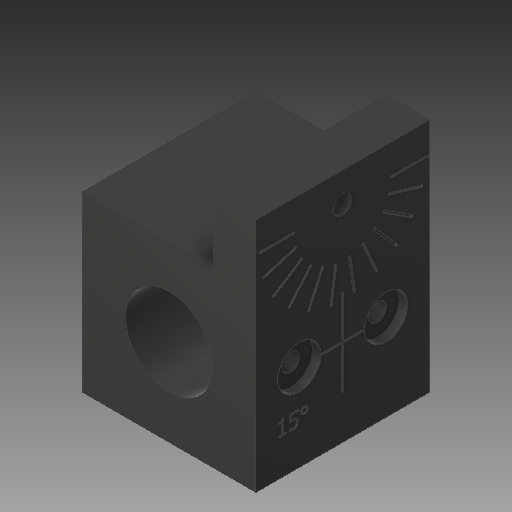
# Autodesk Inventor part: cam_holder_end_part
Saved by Autodesk Inventor 2019 (Build 230136000, 136)
## iProperties
Created: 2024-08-06
Part Number: cam_holder_end_part
Material: Acetalharz, Schwarz
Document SubType Name: Modeling
Designer: nic
Density: 1.425 g/cm^3
Appearance: Glatt - Schwarz
Author: nic
Autodesk Inventor part; units mm, degrees
ref_plane "YZ Plane" through (0, 0, 0) normal (1, 0, 0) x (0, 1, 0)
ref_plane "XY Plane" through (0, 0, 0) normal (0, 0, 1) x (1, 0, 0)
sketch "Skizze1" plane through (0, 0, 0) normal (0, 0, 1) x (1, 0, 0)
  circle A0 centre (0, 0) radius 10.05
  circle A1 centre (0, 0) radius 20
  line L0 (20, 0) -> (10.05, 0)
  line L1 (10.05, 0) -> (10.05, 35)
  line L2 (10.05, 35) -> (20, 35)
  line L3 (20, 35) -> (20, 0)
  dimension "d1" = 40
  dimension "d0" = 20.1
  dimension "d2" = 35
  constraints: 8 end point, 2 coincident, 2 parallel, 1 centre point, 1 horizontal, 1 horizontal alignment, 1 perpendicular, 2 other
  measures "d0" diameter of A0
  measures "d2" distance of L0.end L1.end
extrude "Extrusion1" add sketch "Skizze1" along normal blind 40
sketch "Skizze3" plane through (10.05, 17.2915, 0) normal (-1, 0, 0) x (0, 0, 1)
  line L0 (0, 0) -> (40, 0) construction
  line L1 (40, 17.7085) -> (40, 0) construction
  line L2 (0, 17.7085) -> (40, 17.7085) construction
  line L3 (0, 0) -> (0, 17.7085) construction
  line L4 (0, 17.7085) -> (40, 17.7085) projected
  line L5 (20, 17.7085) -> (20, 7.753)
  line L6 (40, 17.7085) -> (40, 0) projected
  line L7 (40, 10.1178) -> (0, 10.1178)
  point P0 (0, -17.2915)
  point P1 (20, 10.1178)
  constraints: 4 end point, 2 midpoint, 2 point on line, 1 perpendicular, 1 vertical
hole "Bohrung1" at (10.05, 27.4094, 20) direction (1, 0, 0) diameter 4.2 depth 20 tip angle 118 counterbore diameter 8 counterbore depth 3 clearance for "Zylinderschraube mit Schlitz DIN 84" size "M4" standard "DIN"
ref_plane "Arbeitsebene1" through (0, -20, 0) normal (0, 1, 0) x (-1, 0, 0)
sketch "Skizze6" plane through (10.05, 17.2915, 0) normal (-1, 0, 0) x (0, 0, 1)
  circle A0 centre (20, 10.1178) radius 2.1 projected
  circle A1 centre (20, 10.1178) radius 4
  circle A2 centre (20, 10.1178) radius 2.05
  point P0 (0, -17.2915)
  dimension "d37" = 4.1
  constraints: 2 centre point, 2 coincident
  measures "d37" diameter of A2
extrude "Extrusion4" add sketch "Skizze6" against normal up to surface (3 mm away) contours A1
sketch "Skizze15" plane through (0, 0, 0) normal (0, 0, -1) x (-1, 0, 0)
  circle A0 centre (0, 0) radius 10.1
  dimension "d75" = 20.2
  constraints: 1 centre point, 1 coincident
  measures "d75" diameter of A0
extrude "Extrusion14" cut sketch "Skizze15" against normal through all
sketch "Skizze17" plane through (0, 0, 0) normal (0, 0, -1) x (-1, 0, 0)
  line L0 (-20, -20) -> (20, -20)
  line L1 (20, -20) -> (20, 20)
  line L2 (20, 20) -> (-20, 20)
  line L3 (-20, 20) -> (-20, -20)
  line L4 (-20, -20) -> (20, 20) construction
  line L5 (20, -20) -> (-20, 20) construction
  circle A0 centre (0, 0) radius 10.1
  dimension "d82" = 40
  dimension "d83" = 40
  constraints: 12 end point, 2 midpoint, 2 parallel, 1 centre point, 1 coincident, 1 horizontal, 1 perpendicular
  measures "d82" distance of L2.end L1.end
  measures "d83" distance of L1.end L0.end
extrude "Extrusion16" add sketch "Skizze17" against normal up to surface (40 mm away)
sketch "Skizze18" plane through (0, 0, 0) normal (0, 0, -1) x (-1, 0, 0)
  circle A0 centre (0, 0) radius 10.1 construction
  line L0 (7.6, 0.25) -> (12.6, 0.25)
  line L1 (12.6, 0.25) -> (12.6, -0.25)
  line L2 (12.6, -0.25) -> (7.6, -0.25)
  line L3 (7.6, -0.25) -> (7.6, 0.25)
  circle A1 centre (0, 0) radius 10.1 construction
  line L4 (7.6, 0.25) -> (12.6, -0.25) construction
  line L5 (12.6, 0.25) -> (7.6, -0.25) construction
  line L6 (7.4411, 1.5659) -> (12.3652, 2.4342)
  line L7 (12.3652, 2.4342) -> (12.452, 1.9418)
  line L8 (12.452, 1.9418) -> (7.528, 1.0735)
  line L9 (7.528, 1.0735) -> (7.4411, 1.5659)
  line L10 (7.4411, 1.5659) -> (12.452, 1.9418) construction
  line L11 (12.3652, 2.4342) -> (7.528, 1.0735) construction
  line L12 (7.0562, 2.8343) -> (11.7546, 4.5444)
  line L13 (11.7546, 4.5444) -> (11.9256, 4.0745)
  line L14 (11.9256, 4.0745) -> (7.2272, 2.3644)
  line L15 (7.2272, 2.3644) -> (7.0562, 2.8343)
  line L16 (7.0562, 2.8343) -> (11.9256, 4.0745) construction
  line L17 (11.7546, 4.5444) -> (7.2272, 2.3644) construction
  line L18 (6.4568, 4.0165) -> (10.7869, 6.5165)
  line L19 (10.7869, 6.5165) -> (11.0369, 6.0835)
  line L20 (11.0369, 6.0835) -> (6.7068, 3.5835)
  line L21 (6.7068, 3.5835) -> (6.4568, 4.0165)
  line L22 (6.4568, 4.0165) -> (11.0369, 6.0835) construction
  line L23 (10.7869, 6.5165) -> (6.7068, 3.5835) construction
  line L24 (5.6612, 5.0767) -> (9.4915, 8.2906)
  line L25 (9.4915, 8.2906) -> (9.8129, 7.9076)
  line L26 (9.8129, 7.9076) -> (5.9826, 4.6937)
  line L27 (5.9826, 4.6937) -> (5.6612, 5.0767)
  line L28 (5.6612, 5.0767) -> (9.8129, 7.9076) construction
  line L29 (9.4915, 8.2906) -> (5.9826, 4.6937) construction
  line L30 (4.6937, 5.9826) -> (7.9076, 9.8129)
  line L31 (7.9076, 9.8129) -> (8.2906, 9.4915)
  line L32 (8.2906, 9.4915) -> (5.0767, 5.6612)
  line L33 (5.0767, 5.6612) -> (4.6937, 5.9826)
  line L34 (4.6937, 5.9826) -> (8.2906, 9.4915) construction
  line L35 (7.9076, 9.8129) -> (5.0767, 5.6612) construction
  line L36 (3.5835, 6.7068) -> (6.0835, 11.0369)
  line L37 (6.0835, 11.0369) -> (6.5165, 10.7869)
  line L38 (6.5165, 10.7869) -> (4.0165, 6.4568)
  line L39 (4.0165, 6.4568) -> (3.5835, 6.7068)
  line L40 (3.5835, 6.7068) -> (6.5165, 10.7869) construction
  line L41 (6.0835, 11.0369) -> (4.0165, 6.4568) construction
  line L42 (2.3644, 7.2272) -> (4.0745, 11.9256)
  line L43 (4.0745, 11.9256) -> (4.5444, 11.7546)
  line L44 (4.5444, 11.7546) -> (2.8343, 7.0562)
  line L45 (2.8343, 7.0562) -> (2.3644, 7.2272)
  line L46 (2.3644, 7.2272) -> (4.5444, 11.7546) construction
  line L47 (4.0745, 11.9256) -> (2.8343, 7.0562) construction
  line L48 (1.0735, 7.528) -> (1.9418, 12.452)
  line L49 (1.9418, 12.452) -> (2.4342, 12.3652)
  line L50 (2.4342, 12.3652) -> (1.5659, 7.4411)
  line L51 (1.5659, 7.4411) -> (1.0735, 7.528)
  line L52 (1.0735, 7.528) -> (2.4342, 12.3652) construction
  line L53 (1.9418, 12.452) -> (1.5659, 7.4411) construction
  line L54 (-0.25, 7.6) -> (-0.25, 12.6)
  line L55 (-0.25, 12.6) -> (0.25, 12.6)
  line L56 (0.25, 12.6) -> (0.25, 7.6)
  line L57 (0.25, 7.6) -> (-0.25, 7.6)
  line L58 (-0.25, 7.6) -> (0.25, 12.6) construction
  line L59 (-0.25, 12.6) -> (0.25, 7.6) construction
  line L60 (-1.5659, 7.4411) -> (-2.4342, 12.3652)
  line L61 (-2.4342, 12.3652) -> (-1.9418, 12.452)
  line L62 (-1.9418, 12.452) -> (-1.0735, 7.528)
  line L63 (-1.0735, 7.528) -> (-1.5659, 7.4411)
  line L64 (-1.5659, 7.4411) -> (-1.9418, 12.452) construction
  line L65 (-2.4342, 12.3652) -> (-1.0735, 7.528) construction
  line L66 (-2.8343, 7.0562) -> (-4.5444, 11.7546)
  line L67 (-4.5444, 11.7546) -> (-4.0745, 11.9256)
  line L68 (-4.0745, 11.9256) -> (-2.3644, 7.2272)
  line L69 (-2.3644, 7.2272) -> (-2.8343, 7.0562)
  line L70 (-2.8343, 7.0562) -> (-4.0745, 11.9256) construction
  line L71 (-4.5444, 11.7546) -> (-2.3644, 7.2272) construction
  line L72 (-4.0165, 6.4568) -> (-6.5165, 10.7869)
  line L73 (-6.5165, 10.7869) -> (-6.0835, 11.0369)
  line L74 (-6.0835, 11.0369) -> (-3.5835, 6.7068)
  line L75 (-3.5835, 6.7068) -> (-4.0165, 6.4568)
  line L76 (-4.0165, 6.4568) -> (-6.0835, 11.0369) construction
  line L77 (-6.5165, 10.7869) -> (-3.5835, 6.7068) construction
  line L78 (-5.0767, 5.6612) -> (-8.2906, 9.4915)
  line L79 (-8.2906, 9.4915) -> (-7.9076, 9.8129)
  line L80 (-7.9076, 9.8129) -> (-4.6937, 5.9826)
  line L81 (-4.6937, 5.9826) -> (-5.0767, 5.6612)
  line L82 (-5.0767, 5.6612) -> (-7.9076, 9.8129) construction
  line L83 (-8.2906, 9.4915) -> (-4.6937, 5.9826) construction
  line L84 (-5.9826, 4.6937) -> (-9.8129, 7.9076)
  line L85 (-9.8129, 7.9076) -> (-9.4915, 8.2906)
  line L86 (-9.4915, 8.2906) -> (-5.6612, 5.0767)
  line L87 (-5.6612, 5.0767) -> (-5.9826, 4.6937)
  line L88 (-5.9826, 4.6937) -> (-9.4915, 8.2906) construction
  line L89 (-9.8129, 7.9076) -> (-5.6612, 5.0767) construction
  line L90 (-6.7068, 3.5835) -> (-11.0369, 6.0835)
  line L91 (-11.0369, 6.0835) -> (-10.7869, 6.5165)
  line L92 (-10.7869, 6.5165) -> (-6.4568, 4.0165)
  line L93 (-6.4568, 4.0165) -> (-6.7068, 3.5835)
  line L94 (-6.7068, 3.5835) -> (-10.7869, 6.5165) construction
  line L95 (-11.0369, 6.0835) -> (-6.4568, 4.0165) construction
  line L96 (-7.2272, 2.3644) -> (-11.9256, 4.0745)
  line L97 (-11.9256, 4.0745) -> (-11.7546, 4.5444)
  line L98 (-11.7546, 4.5444) -> (-7.0562, 2.8343)
  line L99 (-7.0562, 2.8343) -> (-7.2272, 2.3644)
  line L100 (-7.2272, 2.3644) -> (-11.7546, 4.5444) construction
  line L101 (-11.9256, 4.0745) -> (-7.0562, 2.8343) construction
  line L102 (-7.528, 1.0735) -> (-12.452, 1.9418)
  line L103 (-12.452, 1.9418) -> (-12.3652, 2.4342)
  line L104 (-12.3652, 2.4342) -> (-7.4411, 1.5659)
  line L105 (-7.4411, 1.5659) -> (-7.528, 1.0735)
  line L106 (-7.528, 1.0735) -> (-12.3652, 2.4342) construction
  line L107 (-12.452, 1.9418) -> (-7.4411, 1.5659) construction
  line L108 (-7.6, -0.25) -> (-12.6, -0.25)
  line L109 (-12.6, -0.25) -> (-12.6, 0.25)
  line L110 (-12.6, 0.25) -> (-7.6, 0.25)
  line L111 (-7.6, 0.25) -> (-7.6, -0.25)
  line L112 (-7.6, -0.25) -> (-12.6, 0.25) construction
  line L113 (-12.6, -0.25) -> (-7.6, 0.25) construction
  line L114 (-7.4411, -1.5659) -> (-12.3652, -2.4342)
  line L115 (-12.3652, -2.4342) -> (-12.452, -1.9418)
  line L116 (-12.452, -1.9418) -> (-7.528, -1.0735)
  line L117 (-7.528, -1.0735) -> (-7.4411, -1.5659)
  line L118 (-7.4411, -1.5659) -> (-12.452, -1.9418) construction
  line L119 (-12.3652, -2.4342) -> (-7.528, -1.0735) construction
  line L120 (-7.0562, -2.8343) -> (-11.7546, -4.5444)
  line L121 (-11.7546, -4.5444) -> (-11.9256, -4.0745)
  line L122 (-11.9256, -4.0745) -> (-7.2272, -2.3644)
  line L123 (-7.2272, -2.3644) -> (-7.0562, -2.8343)
  line L124 (-7.0562, -2.8343) -> (-11.9256, -4.0745) construction
  line L125 (-11.7546, -4.5444) -> (-7.2272, -2.3644) construction
  line L126 (-6.4568, -4.0165) -> (-10.7869, -6.5165)
  line L127 (-10.7869, -6.5165) -> (-11.0369, -6.0835)
  line L128 (-11.0369, -6.0835) -> (-6.7068, -3.5835)
  line L129 (-6.7068, -3.5835) -> (-6.4568, -4.0165)
  line L130 (-6.4568, -4.0165) -> (-11.0369, -6.0835) construction
  line L131 (-10.7869, -6.5165) -> (-6.7068, -3.5835) construction
  line L132 (-5.6612, -5.0767) -> (-9.4915, -8.2906)
  line L133 (-9.4915, -8.2906) -> (-9.8129, -7.9076)
  line L134 (-9.8129, -7.9076) -> (-5.9826, -4.6937)
  line L135 (-5.9826, -4.6937) -> (-5.6612, -5.0767)
  line L136 (-5.6612, -5.0767) -> (-9.8129, -7.9076) construction
  line L137 (-9.4915, -8.2906) -> (-5.9826, -4.6937) construction
  line L138 (-4.6937, -5.9826) -> (-7.9076, -9.8129)
  line L139 (-7.9076, -9.8129) -> (-8.2906, -9.4915)
  line L140 (-8.2906, -9.4915) -> (-5.0767, -5.6612)
  line L141 (-5.0767, -5.6612) -> (-4.6937, -5.9826)
  line L142 (-4.6937, -5.9826) -> (-8.2906, -9.4915) construction
  line L143 (-7.9076, -9.8129) -> (-5.0767, -5.6612) construction
  line L144 (-3.5835, -6.7068) -> (-6.0835, -11.0369)
  line L145 (-6.0835, -11.0369) -> (-6.5165, -10.7869)
  line L146 (-6.5165, -10.7869) -> (-4.0165, -6.4568)
  line L147 (-4.0165, -6.4568) -> (-3.5835, -6.7068)
  line L148 (-3.5835, -6.7068) -> (-6.5165, -10.7869) construction
  line L149 (-6.0835, -11.0369) -> (-4.0165, -6.4568) construction
  line L150 (-2.3644, -7.2272) -> (-4.0745, -11.9256)
  line L151 (-4.0745, -11.9256) -> (-4.5444, -11.7546)
  line L152 (-4.5444, -11.7546) -> (-2.8343, -7.0562)
  line L153 (-2.8343, -7.0562) -> (-2.3644, -7.2272)
  line L154 (-2.3644, -7.2272) -> (-4.5444, -11.7546) construction
  line L155 (-4.0745, -11.9256) -> (-2.8343, -7.0562) construction
  line L156 (-1.0735, -7.528) -> (-1.9418, -12.452)
  line L157 (-1.9418, -12.452) -> (-2.4342, -12.3652)
  line L158 (-2.4342, -12.3652) -> (-1.5659, -7.4411)
  line L159 (-1.5659, -7.4411) -> (-1.0735, -7.528)
  line L160 (-1.0735, -7.528) -> (-2.4342, -12.3652) construction
  line L161 (-1.9418, -12.452) -> (-1.5659, -7.4411) construction
  line L162 (0.25, -7.6) -> (0.25, -12.6)
  line L163 (0.25, -12.6) -> (-0.25, -12.6)
  line L164 (-0.25, -12.6) -> (-0.25, -7.6)
  line L165 (-0.25, -7.6) -> (0.25, -7.6)
  line L166 (0.25, -7.6) -> (-0.25, -12.6) construction
  line L167 (0.25, -12.6) -> (-0.25, -7.6) construction
  line L168 (1.5659, -7.4411) -> (2.4342, -12.3652)
  line L169 (2.4342, -12.3652) -> (1.9418, -12.452)
  line L170 (1.9418, -12.452) -> (1.0735, -7.528)
  line L171 (1.0735, -7.528) -> (1.5659, -7.4411)
  line L172 (1.5659, -7.4411) -> (1.9418, -12.452) construction
  line L173 (2.4342, -12.3652) -> (1.0735, -7.528) construction
  line L174 (2.8343, -7.0562) -> (4.5444, -11.7546)
  line L175 (4.5444, -11.7546) -> (4.0745, -11.9256)
  line L176 (4.0745, -11.9256) -> (2.3644, -7.2272)
  line L177 (2.3644, -7.2272) -> (2.8343, -7.0562)
  line L178 (2.8343, -7.0562) -> (4.0745, -11.9256) construction
  line L179 (4.5444, -11.7546) -> (2.3644, -7.2272) construction
  line L180 (4.0165, -6.4568) -> (6.5165, -10.7869)
  line L181 (6.5165, -10.7869) -> (6.0835, -11.0369)
  line L182 (6.0835, -11.0369) -> (3.5835, -6.7068)
  line L183 (3.5835, -6.7068) -> (4.0165, -6.4568)
  line L184 (4.0165, -6.4568) -> (6.0835, -11.0369) construction
  line L185 (6.5165, -10.7869) -> (3.5835, -6.7068) construction
  line L186 (5.0767, -5.6612) -> (8.2906, -9.4915)
  line L187 (8.2906, -9.4915) -> (7.9076, -9.8129)
  line L188 (7.9076, -9.8129) -> (4.6937, -5.9826)
  line L189 (4.6937, -5.9826) -> (5.0767, -5.6612)
  line L190 (5.0767, -5.6612) -> (7.9076, -9.8129) construction
  line L191 (8.2906, -9.4915) -> (4.6937, -5.9826) construction
  line L192 (5.9826, -4.6937) -> (9.8129, -7.9076)
  line L193 (9.8129, -7.9076) -> (9.4915, -8.2906)
  line L194 (9.4915, -8.2906) -> (5.6612, -5.0767)
  line L195 (5.6612, -5.0767) -> (5.9826, -4.6937)
  line L196 (5.9826, -4.6937) -> (9.4915, -8.2906) construction
  line L197 (9.8129, -7.9076) -> (5.6612, -5.0767) construction
  line L198 (6.7068, -3.5835) -> (11.0369, -6.0835)
  line L199 (11.0369, -6.0835) -> (10.7869, -6.5165)
  line L200 (10.7869, -6.5165) -> (6.4568, -4.0165)
  line L201 (6.4568, -4.0165) -> (6.7068, -3.5835)
  line L202 (6.7068, -3.5835) -> (10.7869, -6.5165) construction
  line L203 (11.0369, -6.0835) -> (6.4568, -4.0165) construction
  line L204 (7.2272, -2.3644) -> (11.9256, -4.0745)
  line L205 (11.9256, -4.0745) -> (11.7546, -4.5444)
  line L206 (11.7546, -4.5444) -> (7.0562, -2.8343)
  line L207 (7.0562, -2.8343) -> (7.2272, -2.3644)
  line L208 (7.2272, -2.3644) -> (11.7546, -4.5444) construction
  line L209 (11.9256, -4.0745) -> (7.0562, -2.8343) construction
  line L210 (7.528, -1.0735) -> (12.452, -1.9418)
  line L211 (12.452, -1.9418) -> (12.3652, -2.4342)
  line L212 (12.3652, -2.4342) -> (7.4411, -1.5659)
  line L213 (7.4411, -1.5659) -> (7.528, -1.0735)
  line L214 (7.528, -1.0735) -> (12.3652, -2.4342) construction
  line L215 (12.452, -1.9418) -> (7.4411, -1.5659) construction
  line L216 (-15, 0.25) -> (15, 0.25)
  line L217 (15, 0.25) -> (15, -0.25)
  line L218 (15, -0.25) -> (-15, -0.25)
  line L219 (-15, -0.25) -> (-15, 0.25)
  line L220 (-15, 0.25) -> (15, -0.25) construction
  line L221 (15, 0.25) -> (-15, -0.25) construction
  point P0 (10.1, 0)
  point P1 (9.9466, 1.7538)
  point P2 (9.4909, 3.4544)
  point P3 (8.7469, 5.05)
  point P4 (7.737, 6.4922)
  point P5 (6.4922, 7.737)
  point P6 (5.05, 8.7469)
  point P7 (3.4544, 9.4909)
  point P8 (1.7538, 9.9466)
  point P9 (0, 10.1)
  point P10 (-1.7538, 9.9466)
  point P11 (-3.4544, 9.4909)
  point P12 (-5.05, 8.7469)
  point P13 (-6.4922, 7.737)
  point P14 (-7.737, 6.4922)
  point P15 (-8.7469, 5.05)
  point P16 (-9.4909, 3.4544)
  point P17 (-9.9466, 1.7538)
  point P18 (-10.1, 0)
  point P19 (-9.9466, -1.7538)
  point P20 (-9.4909, -3.4544)
  point P21 (-8.7469, -5.05)
  point P22 (-7.737, -6.4922)
  point P23 (-6.4922, -7.737)
  point P24 (-5.05, -8.7469)
  point P25 (-3.4544, -9.4909)
  point P26 (-1.7538, -9.9466)
  point P27 (0, -10.1)
  point P28 (1.7538, -9.9466)
  point P29 (3.4544, -9.4909)
  point P30 (5.05, -8.7469)
  point P31 (6.4922, -7.737)
  point P32 (7.737, -6.4922)
  point P33 (8.7469, -5.05)
  point P34 (9.4909, -3.4544)
  point P35 (9.9466, -1.7538)
  dimension "d86" = 5
  dimension "d87" = 0.5
  dimension "d90" = 360
  dimension "d92" = 30
  dimension "d93" = 0.5
  constraints: 444 end point, 74 midpoint, 4 parallel, 2 horizontal, 2 perpendicular, 1 horizontal alignment, 398 other
  measures "d86" distance of L1.end L2.end
  measures "d87" distance of L0.end L1.end
  measures "d92" distance of L217.end L218.end
  measures "d93" distance of L216.end L217.end
extrude "Extrusion17" cut sketch "Skizze18" against normal blind 0.5
sketch "Skizze19" plane through (20, 35, 40) normal (1, 0, 0) x (0, 0, -1)
  line L0 (40, -35) -> (30, -35)
  line L1 (0, -55) -> (0, -15) projected
  line L2 (39.5, -45.1) -> (0, -45.1) projected
  line L3 (0, -45.1) -> (10, -45.1)
  point P0 (10, -35)
  dimension "d96" = 10
  dimension "d97" = 10
  constraints: 4 end point, 3 point on line, 1 coincident, 1 perpendicular
  measures "d96" distance of L0.start L0.end
  measures "d97" distance of L3.start L3.end
hole "Bohrung3" at (20, 0, 10) at (20, 0, 30) direction (-1, 0, 0) diameter 4.2 depth 20 tip angle 118 counterbore diameter 10 counterbore depth 2
sketch "Skizze20" plane through (20, 35, 40) normal (1, 0, 0) x (0, 0, -1)
  circle A0 centre (20, -7.5906) radius 2.1 construction
  circle A1 centre (30, -35) radius 5 construction
  circle A2 centre (30, -35) radius 2.1 construction
  circle A3 centre (10, -35) radius 2.1 construction
  line L0 (30, -35) -> (10, -35) construction
  line L1 (20, -7.5906) -> (20, -35) construction
  line L2 (20.25, -25) -> (19.75, -25)
  line L3 (19.75, -25) -> (19.75, -45)
  line L4 (19.75, -45) -> (20.25, -45)
  line L5 (20.25, -45) -> (20.25, -25)
  line L6 (20.25, -25) -> (19.75, -45) construction
  line L7 (19.75, -25) -> (20.25, -45) construction
  line L8 (14.9937, -34.75) -> (25.0063, -34.75)
  line L9 (25.0063, -34.75) -> (25.0063, -35.25)
  line L10 (25.0063, -35.25) -> (14.9937, -35.25)
  line L11 (14.9937, -35.25) -> (14.9937, -34.75)
  line L12 (14.9937, -34.75) -> (25.0063, -35.25) construction
  line L13 (25.0063, -34.75) -> (14.9937, -35.25) construction
  point P0 (40, -35)
  dimension "d105" = 0.5
  dimension "d106" = 20
  dimension "d107" = 0.5
  constraints: 28 end point, 5 midpoint, 4 parallel, 3 horizontal, 2 perpendicular, 2 other
  measures "d105" distance of L4.end L3.end
  measures "d106" distance of L3.end L2.end
  measures "d107" distance of L8.end L9.end
extrude "Extrusion18" cut sketch "Skizze20" against normal blind 0.5
sketch "Skizze23" plane through (20, 35, 40) normal (1, 0, 0) x (0, 0, -1)
  circle A0 centre (20, -7.5906) radius 2.1 projected
  line L0 (20, -7.5906) -> (20, -0.5906)
  line L1 (40, -0.5906) -> (-0.1444, -0.5906)
  line L2 (-0.1444, -0.5906) -> (-0.1444, 3.8544)
  line L3 (-0.1444, 3.8544) -> (40, 3.8544)
  line L4 (40, 3.8544) -> (40, -0.5906)
  point P0 (40, -35)
  dimension "d122" = 7
  constraints: 10 end point, 2 parallel, 1 horizontal, 1 perpendicular, 1 vertical
  measures "d122" distance of L0.start L0.end
extrude "Extrusion21" cut sketch "Skizze23" against normal through all contours L1 L2 L3 L4
sketch "Skizze24" plane through (20, -20, 40) normal (1, 0, 0) x (0, 0, -1)
  circle A0 centre (20, 47.4094) radius 2.05 projected
  line L0 (39.084, 47.1594) -> (31.084, 47.1594)
  line L1 (31.084, 47.1594) -> (31.084, 47.6594)
  line L2 (31.084, 47.6594) -> (39.084, 47.6594)
  line L3 (39.084, 47.6594) -> (39.084, 47.1594)
  line L4 (39.084, 47.1594) -> (31.084, 47.6594) construction
  line L5 (31.084, 47.1594) -> (39.084, 47.6594) construction
  line L6 (38.2405, 41.7929) -> (30.5646, 44.0468)
  line L7 (30.5646, 44.0468) -> (30.7054, 44.5265)
  line L8 (30.7054, 44.5265) -> (38.3814, 42.2727)
  line L9 (38.3814, 42.2727) -> (38.2405, 41.7929)
  line L10 (38.2405, 41.7929) -> (30.7054, 44.5265) construction
  line L11 (30.5646, 44.0468) -> (38.3814, 42.2727) construction
  line L12 (35.9193, 36.8815) -> (29.1893, 41.2066)
  line L13 (29.1893, 41.2066) -> (29.4596, 41.6272)
  line L14 (29.4596, 41.6272) -> (36.1896, 37.3021)
  line L15 (36.1896, 37.3021) -> (35.9193, 36.8815)
  line L16 (35.9193, 36.8815) -> (29.4596, 41.6272) construction
  line L17 (29.1893, 41.2066) -> (36.1896, 37.3021) construction
  line L18 (32.3084, 32.8229) -> (27.0695, 38.8689)
  line L19 (27.0695, 38.8689) -> (27.4474, 39.1964)
  line L20 (27.4474, 39.1964) -> (32.6863, 33.1504)
  line L21 (32.6863, 33.1504) -> (32.3084, 32.8229)
  line L22 (32.3084, 32.8229) -> (27.4474, 39.1964) construction
  line L23 (27.0695, 38.8689) -> (32.6863, 33.1504) construction
  line L24 (27.7004, 29.9461) -> (24.377, 37.2232)
  line L25 (24.377, 37.2232) -> (24.8319, 37.4309)
  line L26 (24.8319, 37.4309) -> (28.1552, 30.1538)
  line L27 (28.1552, 30.1538) -> (27.7004, 29.9461)
  line L28 (27.7004, 29.9461) -> (24.8319, 37.4309) construction
  line L29 (24.377, 37.2232) -> (28.1552, 30.1538) construction
  line L30 (22.4685, 28.4841) -> (21.33, 36.4026)
  line L31 (21.33, 36.4026) -> (21.8249, 36.4738)
  line L32 (21.8249, 36.4738) -> (22.9634, 28.5552)
  line L33 (22.9634, 28.5552) -> (22.4685, 28.4841)
  line L34 (22.4685, 28.4841) -> (21.8249, 36.4738) construction
  line L35 (21.33, 36.4026) -> (22.9634, 28.5552) construction
  line L36 (17.0366, 28.5552) -> (18.1751, 36.4738)
  line L37 (18.1751, 36.4738) -> (18.67, 36.4026)
  line L38 (18.67, 36.4026) -> (17.5315, 28.4841)
  line L39 (17.5315, 28.4841) -> (17.0366, 28.5552)
  line L40 (17.0366, 28.5552) -> (18.67, 36.4026) construction
  line L41 (18.1751, 36.4738) -> (17.5315, 28.4841) construction
  line L42 (11.8448, 30.1538) -> (15.1681, 37.4309)
  line L43 (15.1681, 37.4309) -> (15.623, 37.2232)
  line L44 (15.623, 37.2232) -> (12.2996, 29.9461)
  line L45 (12.2996, 29.9461) -> (11.8448, 30.1538)
  line L46 (11.8448, 30.1538) -> (15.623, 37.2232) construction
  line L47 (15.1681, 37.4309) -> (12.2996, 29.9461) construction
  line L48 (7.3137, 33.1504) -> (12.5526, 39.1964)
  line L49 (12.5526, 39.1964) -> (12.9305, 38.8689)
  line L50 (12.9305, 38.8689) -> (7.6916, 32.8229)
  line L51 (7.6916, 32.8229) -> (7.3137, 33.1504)
  line L52 (7.3137, 33.1504) -> (12.9305, 38.8689) construction
  line L53 (12.5526, 39.1964) -> (7.6916, 32.8229) construction
  line L54 (3.8104, 37.3021) -> (10.5404, 41.6272)
  line L55 (10.5404, 41.6272) -> (10.8107, 41.2066)
  line L56 (10.8107, 41.2066) -> (4.0807, 36.8815)
  line L57 (4.0807, 36.8815) -> (3.8104, 37.3021)
  line L58 (3.8104, 37.3021) -> (10.8107, 41.2066) construction
  line L59 (10.5404, 41.6272) -> (4.0807, 36.8815) construction
  line L60 (1.6186, 42.2727) -> (9.2946, 44.5265)
  line L61 (9.2946, 44.5265) -> (9.4354, 44.0468)
  line L62 (9.4354, 44.0468) -> (1.7595, 41.7929)
  line L63 (1.7595, 41.7929) -> (1.6186, 42.2727)
  line L64 (1.6186, 42.2727) -> (9.4354, 44.0468) construction
  line L65 (9.2946, 44.5265) -> (1.7595, 41.7929) construction
  line L66 (0.916, 47.6594) -> (8.916, 47.6594)
  line L67 (8.916, 47.6594) -> (8.916, 47.1594)
  line L68 (8.916, 47.1594) -> (0.916, 47.1594)
  line L69 (0.916, 47.1594) -> (0.916, 47.6594)
  line L70 (0.916, 47.6594) -> (8.916, 47.1594) construction
  line L71 (8.916, 47.6594) -> (0.916, 47.1594) construction
  line L72 (4.7436, 11.7718) -> (15.9499, 11.7718) construction
  line L73 (15.9499, 11.7718) -> (15.9499, 2.8068) construction
  line L74 (15.9499, 2.8068) -> (4.7436, 2.8068) construction
  line L75 (4.7436, 2.8068) -> (4.7436, 11.7718) construction
  line L76 (6.9815, 8.2122) -> (5.274, 8.2122)
  line L77 (5.274, 8.2122) -> (5.274, 8.5696)
  line L78 (5.274, 8.5696) -> (5.9093, 8.5696)
  line L79 (5.9093, 8.5696) -> (5.9093, 10.9152)
  line L80 (5.9093, 10.9152) -> (5.274, 10.9152)
  line L81 (5.274, 10.9152) -> (5.274, 11.2357)
  spline S0 degree 2 poles (5.274, 11.2357) (5.6342, 11.2357) (5.9746, 11.4399) (5.9973, 11.7236) knots 0 0 0 1 2 2 2
  line L82 (5.9973, 11.7236) -> (6.3603, 11.7236)
  line L83 (6.3603, 11.7236) -> (6.3603, 8.5696)
  line L84 (6.3603, 8.5696) -> (6.9815, 8.5696)
  line L85 (6.9815, 8.5696) -> (6.9815, 8.2122)
  spline S1 degree 2 poles (9.7469, 9.3241) (9.7469, 9.0716) (9.5852, 8.6405) (9.4377, 8.4817) knots 0 0 0 1 2 2 2
  spline S2 degree 2 poles (9.4377, 8.4817) (9.2902, 8.3228) (8.8506, 8.1385) (8.5783, 8.1385) knots 0 0 0 1 2 2 2
  spline S3 degree 2 poles (8.5783, 8.1385) (8.3287, 8.1385) (7.8409, 8.2491) (7.6622, 8.337) knots 0 0 0 1 2 2 2
  line L86 (7.6622, 8.337) -> (7.6622, 8.8334)
  line L87 (7.6622, 8.8334) -> (7.6962, 8.8334)
  spline S4 degree 2 poles (7.6962, 8.8334) (7.7501, 8.7937) (7.9515, 8.6916) (8.0734, 8.6462) knots 0 0 0 1 2 2 2
  spline S5 degree 2 poles (8.0734, 8.6462) (8.2124, 8.598) (8.4422, 8.5441) (8.5868, 8.5441) knots 0 0 0 1 2 2 2
  spline S6 degree 2 poles (8.5868, 8.5441) (8.7286, 8.5441) (8.9952, 8.6462) (9.0917, 8.7568) knots 0 0 0 1 2 2 2
  spline S7 degree 2 poles (9.0917, 8.7568) (9.1796, 8.8617) (9.2704, 9.1397) (9.2704, 9.3269) knots 0 0 0 1 2 2 2
  spline S8 degree 2 poles (9.2704, 9.3269) (9.2704, 9.5141) (9.1682, 9.7523) (9.0718, 9.8318) knots 0 0 0 1 2 2 2
  spline S9 degree 2 poles (9.0718, 9.8318) (8.9725, 9.9197) (8.6776, 9.9934) (8.4989, 9.9934) knots 0 0 0 1 2 2 2
  spline S10 degree 2 poles (8.4989, 9.9934) (8.306, 9.9934) (7.9231, 9.9339) (7.8068, 9.9083) knots 0 0 0 1 2 2 2
  line L88 (7.8068, 9.9083) -> (7.8068, 11.7122)
  line L89 (7.8068, 11.7122) -> (9.727, 11.7122)
  line L90 (9.727, 11.7122) -> (9.727, 11.301)
  line L91 (9.727, 11.301) -> (8.2578, 11.301)
  line L92 (8.2578, 11.301) -> (8.2578, 10.3678)
  spline S11 degree 2 poles (8.2578, 10.3678) (8.3429, 10.3792) (8.5074, 10.3877) (8.5755, 10.3877) knots 0 0 0 1 2 2 2
  spline S12 degree 2 poles (8.5755, 10.3877) (8.8449, 10.3877) (9.2165, 10.2997) (9.3866, 10.1693) knots 0 0 0 1 2 2 2
  spline S13 degree 2 poles (9.3866, 10.1693) (9.5597, 10.0388) (9.7469, 9.6417) (9.7469, 9.3241) knots 0 0 0 1 2 2 2
  spline S14 degree 2 poles (12.0244, 10.8784) (12.0244, 10.5011) (11.5082, 9.9849) (11.131, 9.9849) knots 0 0 0 1 2 2 2
  spline S15 degree 2 poles (11.131, 9.9849) (10.7566, 9.9849) (10.2347, 10.4983) (10.2347, 10.8784) knots 0 0 0 1 2 2 2
  spline S16 degree 2 poles (10.2347, 10.8784) (10.2347, 11.2556) (10.7509, 11.7718) (11.131, 11.7718) knots 0 0 0 1 2 2 2
  spline S17 degree 2 poles (11.131, 11.7718) (11.5082, 11.7718) (12.0244, 11.2556) (12.0244, 10.8784) knots 0 0 0 1 2 2 2
  spline S18 degree 2 poles (11.6557, 10.8784) (11.6557, 11.1053) (11.355, 11.4144) (11.131, 11.4144) knots 0 0 0 1 2 2 2
  spline S19 degree 2 poles (11.131, 11.4144) (10.9041, 11.4144) (10.6034, 11.1053) (10.6034, 10.8784) knots 0 0 0 1 2 2 2
  spline S20 degree 2 poles (10.6034, 10.8784) (10.6034, 10.6486) (10.9097, 10.3423) (11.131, 10.3423) knots 0 0 0 1 2 2 2
  spline S21 degree 2 poles (11.131, 10.3423) (11.355, 10.3423) (11.6557, 10.6543) (11.6557, 10.8784) knots 0 0 0 1 2 2 2
  point P0 (40, 20)
  point P1 (35.084, 47.4094)
  point P2 (34.473, 43.1597)
  point P3 (32.6894, 39.2543)
  point P4 (29.8779, 36.0097)
  point P5 (26.2661, 33.6885)
  point P6 (22.1467, 32.4789)
  point P7 (17.8533, 32.4789)
  point P8 (13.7339, 33.6885)
  point P9 (10.1221, 36.0097)
  point P10 (7.3106, 39.2543)
  point P11 (5.527, 43.1597)
  point P12 (4.916, 47.4094)
  dimension "d125" = 8
  dimension "d126" = 0.5
  dimension "d129" = 180
  constraints: 144 end point, 24 midpoint, 2 parallel, 1 horizontal, 1 perpendicular, 124 other
  measures "d125" distance of L1.end L2.end
  measures "d126" distance of L0.end L1.end
extrude "Extrusion22" cut sketch "Skizze24" against normal blind 0.5 contours L0 L1 L2 L3 | L6 L7 L8 L9 | L12 L13 L14 L15 | L18 L19 L20 L21 | L24 L25 L26 L27 | L30 L31 L32 L33 | L36 L37 L38 L39 | L42 L43 L44 L45 | L48 L49 L50 L51 | L54 L55 L56 L57 | L60 L61 L62 L63 | L66 L67 L68 L69 | L76 L77 L78 L79 L80 L81 S0 L82 L83 L84 L85 | S1 S2 S3 L86 L87 S4 S5 S6 S7 S8 S9 S10 L88 L89 L90 L91 L92 S11 S12 S13 | S14 S15 S16 S17
sketch "Skizze27" plane through (0, 0, 0) normal (0, 0, -1) x (-1, 0, 0)
  line L0 (-0.25, 12.6) -> (-0.25, 10.0969) projected
  line L1 (0.25, 10.0969) -> (0.25, 12.6) projected
  line L2 (-0.25, 10.0969) -> (-0.25, 12.6) projected
  line L3 (20, 20) -> (-10.05, 20) projected
  line L4 (-0.25, 12.6) -> (0.25, 12.6)
  line L5 (0.25, 12.6) -> (0.25, 20)
  line L6 (0.25, 20) -> (-0.25, 20)
  line L7 (-0.25, 20) -> (-0.25, 12.6)
  point P0 (0, 0)
  constraints: 8 end point, 2 parallel, 1 horizontal, 1 perpendicular, 1 point on line, 1 other
extrude "Extrusion23" cut sketch "Skizze27" against normal blind 0.5
sketch "Skizze28" plane through (0, 0, 0) normal (0, 0, -1) x (-1, 0, 0)
  line L0 (-10.05, 29.5094) -> (-10.05, 25.3094) projected
  line L1 (-20, 34.4094) -> (-20, -20) projected
  line L2 (-0.1, 26.9547) -> (-20, 26.9547)
  line L3 (-20, 26.9547) -> (-20, 27.4547)
  line L4 (-20, 27.4547) -> (-0.1, 27.4547)
  line L5 (-0.1, 27.4547) -> (-0.1, 26.9547)
  line L6 (-10.05, 20) -> (-10.05, 34.4094) projected
  line L7 (-0.1, 26.9547) -> (-20, 27.4547) construction
  line L8 (-20, 26.9547) -> (-0.1, 27.4547) construction
  point P0 (0, 0)
  point P1 (-10.05, 27.2047)
  dimension "d135" = 0.5
  constraints: 12 end point, 3 midpoint, 2 parallel, 1 horizontal, 1 perpendicular, 1 point on line
  measures "d135" distance of L2.end L3.end
extrude "Extrusion24" cut sketch "Skizze28" against normal blind 0.5
